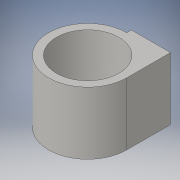
# Autodesk Inventor part: motor spinner
Saved by Autodesk Inventor 2016 (Build 200138000, 138)
## iProperties
Created: 2016-02-23
Part Number: motor spinner
Material: Generic
Document SubType Name: Modeling
Designer: Admin
Density: 1 g/cm^3
Appearance: Default
Author: Admin
Autodesk Inventor part; units mm, degrees
ref_plane "YZ Plane" through (0, 0, 0) normal (1, 0, 0) x (0, 1, 0)
ref_plane "XZ Plane" through (0, 0, 0) normal (0, 1, 0) x (-1, 0, 0)
ref_plane "XY Plane" through (0, 0, 0) normal (0, 0, 1) x (1, 0, 0)
sketch "Sketch1" plane through (0, 0, 0) normal (0, 1, 0) x (-1, 0, 0)
  circle A0 centre (0, 0) radius 12.7
  arc A1 (0, -15.875) -> (-15.875, 0) centre (0, 0) ccw
  line L0 (-15.875, -12.7) -> (-15.875, -17.78)
  line L1 (-15.875, -17.78) -> (0, -17.78)
  line L2 (0, -17.78) -> (0, -12.7)
  line L3 (-15.875, -12.7) -> (-15.875, 0)
  dimension "d0" = 25.4
  dimension "d1" = 31.75
  dimension "d2" = 5.08
  constraints: 8 end point, 2 coincident, 2 point on circle, 1 centre point, 1 parallel, 1 point on line, 1 tangent, 1 vertical alignment, 2 other
  measures "d1" diameter of A1
  measures "d2" distance of L0.end L0.start
extrude "Extrusion1" add sketch "Sketch1" along normal blind 25.4
sketch "Sketch2" plane through (15.875, 0, -17.78) normal (0, 0, -1) x (-1, 0, 0)
  circle A0 centre (7.9375, 12.7) radius 2.54
  line L0 (15.875, 0) -> (15.875, 25.4) projected
  dimension "d5" = 5.08
  dimension "d6" = 7.9375
  constraints: 1 centre point
  measures "d5" diameter of A0
  measures "d6" distance from line of L0 A0.centre
extrude "Extrusion2" cut sketch "Sketch2" against normal blind 13.081
sketch "Sketch3" plane through (15.875, 0, -17.78) normal (0, 0, -1) x (-1, 0, 0)
  circle A0 centre (7.9375, 12.7) radius 3.175
  line L0 (15.875, 0) -> (15.875, 25.4) projected
  dimension "d9" = 6.35
  dimension "d10" = 7.9375
  constraints: 1 centre point
  measures "d9" diameter of A0
  measures "d10" distance from line of L0 A0.centre
extrude "Extrusion3" cut sketch "Sketch3" against normal blind 5.08
body "Solid1"
